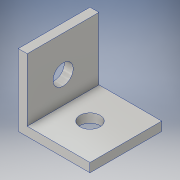
# Autodesk Inventor part: Lbracket
Saved by Autodesk Inventor 2016 (Build 200138000, 138)
## iProperties
Created: 2017-01-27
Part Number: Lbracket
Material: Aluminum 6061
Document SubType Name: Modeling
Designer: hamblettk
Density: 2.7 g/cm^3
Appearance: Aluminum - Flat
Author: hamblettk
Autodesk Inventor part; units mm, degrees
ref_plane "YZ Plane" through (0, 0, 0) normal (1, 0, 0) x (0, 1, 0)
ref_plane "XZ Plane" through (0, 0, 0) normal (0, 1, 0) x (-1, 0, 0)
ref_plane "XY Plane" through (0, 0, 0) normal (0, 0, 1) x (1, 0, 0)
sketch "Sketch1" plane through (0, 0, 0) normal (0, 1, 0) x (-1, 0, 0)
  line L0 (0, 0) -> (25.4, 0)
  line L1 (25.4, 0) -> (25.4, -25.4)
  line L2 (25.4, -25.4) -> (0, -25.4)
  line L3 (0, -25.4) -> (0, 0)
  dimension "d0" = 25.4
  dimension "d1" = 25.4
  constraints: 8 end point, 2 parallel, 1 horizontal, 1 perpendicular
  measures "d0" distance of L1.end L2.end
  measures "d1" distance of L0.end L1.end
extrude "Extrusion1" add sketch "Sketch1" along normal blind 3.175
sketch "Sketch2" plane through (0, 3.175, 0) normal (0, 1, 0) x (1, 0, 0)
  line L0 (-25.4, 25.4) -> (-25.4, 0) projected
  line L1 (-25.4, 0) -> (-22.225, 0)
  line L2 (-22.225, 0) -> (-22.225, 25.4)
  line L3 (-22.225, 25.4) -> (-25.4, 25.4)
  line L4 (-25.4, 25.4) -> (-25.4, 0)
  point P0 (0, 0)
  dimension "d4" = 3.175
  dimension "d5" = 25.4
  constraints: 8 end point, 2 parallel, 1 horizontal, 1 perpendicular
  measures "d4" distance of L3.end L2.end
  measures "d5" distance of L2.end L1.end
extrude "Extrusion2" add sketch "Sketch2" along normal blind 22.225
sketch "Sketch3" plane through (0, 3.175, 0) normal (0, 1, 0) x (1, 0, 0)
  circle A0 centre (-12.7, 12.7) radius 3.5687
  line L0 (0, 25.4) -> (-22.225, 25.4) projected
  line L1 (0, 25.4) -> (0, 0) projected
  dimension "d8" = 7.1374
  dimension "d9" = 12.7
  dimension "d10" = 12.7
  constraints: 1 centre point
  measures "d8" diameter of A0
  measures "d9" distance from line of L0 A0.centre
  measures "d10" distance from line of L1 A0.centre
extrude "Extrusion3" cut sketch "Sketch3" against normal blind 22.225
sketch "Sketch4" plane through (-22.225, 3.175, 0) normal (1, 0, 0) x (0, 0, -1)
  circle A0 centre (12.7, 9.525) radius 3.5687
  line L0 (25.4, 0) -> (25.4, 22.225) projected
  line L1 (0, 22.225) -> (25.4, 22.225) projected
  point P0 (0, -3.175)
  dimension "d13" = 7.1374
  dimension "d14" = 12.7
  dimension "d15" = 12.7
  constraints: 1 centre point
  measures "d13" diameter of A0
  measures "d14" distance from line of L0 A0.centre
  measures "d15" distance from line of L1 A0.centre
extrude "Extrusion4" cut sketch "Sketch4" against normal blind 3.175
body "Solid1"
